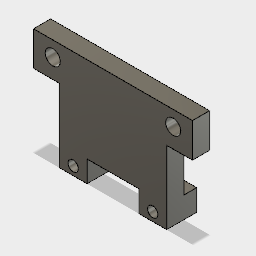
Ir Touch Probe Bracket (Autodesk Fusion 360 design; units mm, degrees)
Autodesk Fusion 360 part; units mm, degrees
sketch "Sketch1" plane through (0, 0, 0) normal (0, 0, 1) x (1, 0, 0)
  line L0 (0, 0) -> (37, 0)
  line L1 (37, 0) -> (37, 8)
  line L2 (37, 8) -> (0, 8)
  line L3 (0, 8) -> (0, 0)
  circle A0 centre (32.5, 4.5) radius 1.75
  circle A1 centre (4.5, 4.5) radius 1.75
  line L4 (16, 8) -> (21, 8)
  line L5 (21, 0) -> (16, 0)
  line L6 (31, -17) -> (24.5, -17)
  line L7 (24.5, -17) -> (24.5, -12)
  line L8 (31, -12) -> (31, -17)
  line L9 (24.5, -12) -> (31, -12)
  line L10 (6, -17) -> (6, -12)
  line L11 (12.5, -17) -> (6, -17)
  line L12 (12.5, -12) -> (12.5, -17)
  line L13 (6, -12) -> (12.5, -12)
  circle A2 centre (27.75, -15) radius 1.2
  circle A3 centre (9.25, -15) radius 1.2
  line L14 (31, -17) -> (6, -17)
  line L15 (6, -17) -> (6, 0)
  line L16 (6, 0) -> (31, 0)
  line L17 (31, 0) -> (31, -17)
  line L18 (12.5, -12) -> (24.5, -12)
  dimension "d1" = 37
  dimension "d2" = 8
  dimension "d3" = 3.5
  dimension "d6" = 3.5
  dimension "d9" = 4.5
  dimension "d10" = 4.5
  dimension "d45" = 6.5
  dimension "d46" = 5
  dimension "d47" = 5
  dimension "d48" = 6.5
  dimension "d49" = 2.4
  dimension "d50" = 2.4
  dimension "d51" = 12
  dimension "d52" = 12
  dimension "d53" = 12
  dimension "d54" = 3.25
  dimension "d55" = 2
  dimension "d56" = 2
  dimension "d57" = 3.25
  dimension "d62" = 25
  dimension "d96" = 4.5
  dimension "d97" = 4.5
  measures "d1" distance of L0.start L0.end
  measures "d2" distance of L0.start L2.end
  measures "d3" diameter of A0
  measures "d6" diameter of A1
  measures "d9" distance of L1 A0.centre
  measures "d10" distance of L3 A1.centre
  measures "d45" distance of L7.end L8.start
  measures "d46" distance of L6.end L7.end
  measures "d47" distance of L10.end L10.start
  measures "d48" distance of L10 L12
  measures "d49" diameter of A2
  measures "d50" diameter of A3
  measures "d51" distance of L0 L9
  measures "d52" distance of L0 L13
  measures "d53" distance of L7 L12
  measures "d54" distance of L10 A3.centre
  measures "d55" distance of L11 A3.centre
  measures "d56" distance of L6 A2.centre
  measures "d57" distance of L7 A2.centre
  measures "d62" distance of L6.start L10.start
  measures "d96" distance of L0 A0.centre
  measures "d97" distance of L0 A1.centre
extrude "Extrude16" add sketch "Sketch1" against normal blind 4 contours L0 L1 L2 L3 L4 L5 L16
extrude "Extrude17" add sketch "Sketch1" against normal blind 4 contours L0 L5 L9 L13 L15 L16 L17 L18
extrude "Extrude18" add sketch "Sketch1" against normal blind 7 contours L6 L7 L8 L9 L14 L17
extrude "Extrude19" add sketch "Sketch1" against normal blind 7 contours L10 L11 L12 L13 L14 L15
